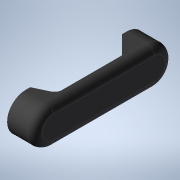
# Autodesk Inventor part: controlbox_handvat
Saved by Autodesk Inventor 2020 (Build 240168000, 168)
## iProperties
Created: 2020-06-02
Part Number: controlbox_handvat
Material: Generic
Document SubType Name: Modeling
Designer: Gebruiker
Density: 1 g/cm^3
Appearance: Default
Author: Gebruiker
Autodesk Inventor part; units mm, degrees
ref_plane "YZ Plane" through (0, 0, 0) normal (1, 0, 0) x (0, 1, 0)
ref_plane "XZ Plane" through (0, 0, 0) normal (0, 1, 0) x (-1, 0, 0)
ref_plane "XY Plane" through (0, 0, 0) normal (0, 0, 1) x (1, 0, 0)
sketch "Sketch1" plane through (0, 0, 0) normal (1, 0, 0) x (0, 1, 0)
  line L0 (10, 37.5) -> (-10, 37.5)
  line L1 (-10, 37.5) -> (-10, -37.5)
  line L2 (-10, -37.5) -> (10, -37.5)
  line L3 (10, -37.5) -> (10, 37.5)
  line L4 (10, 37.5) -> (-10, -37.5) construction
  line L5 (-10, 37.5) -> (10, -37.5) construction
  circle A0 centre (0, 27.5) radius 10
  circle A1 centre (0, -27.5) radius 10
  point P0 (0, 0)
  point P1 (10, -27.5)
  point P2 (10, 27.5)
  point P3 (-10, 27.5)
  point P4 (-10, -27.5)
  dimension "d0" = 20
  dimension "d1" = 75
  dimension "d2" = 20
  dimension "d3" = 20
  dimension "d4" = 55
  constraints: 12 end point, 2 centre point, 2 midpoint, 2 parallel, 1 horizontal, 1 perpendicular, 1 tangent
  measures "d0" distance of L2.end L1.end
  measures "d1" distance of L1.end L0.end
  measures "d2" diameter of A0
  measures "d3" diameter of A1
  measures "d4" distance of A1.centre A0.centre
extrude "Extrusion1" add sketch "Sketch1" against normal blind 15 contours A0 | L3 A1 L1 A0 | A1
sketch "Sketch2" plane through (0, -10, -27.5) normal (0, -1, 0) x (1, 0, 0)
  line L0 (-15, 55) -> (-15, 0) projected
  line L1 (-15, 52.5125) -> (-5.0401, 47.8284)
  line L2 (-5.0401, 47.8284) -> (-5.0401, 7.1716)
  line L3 (-5.0401, 7.1716) -> (-15, 2.4875)
  line L4 (-15, 0) -> (-15, -10) projected
  line L5 (0, 55) -> (0, 65) construction
  line L6 (0, 65) -> (-5.0401, 47.8284) construction
  line L7 (0, -10) -> (0, 0) construction
  line L8 (-5.0401, 7.1716) -> (0, -10) construction
  point P0 (0, 27.5)
  point P1 (-15, 2.4875)
  constraints: 10 end point, 2 equal length, 2 point on line, 1 parallel
extrude "Extrusion2" cut sketch "Sketch2" against normal blind 20
fillet "Fillet1" radius 4 6 edges at (0, -10, 0) (0, 0, -37.5) (0, 10, 0) (0, 0, 37.5) (-5.0401, 0, -20.3284) (-5.0401, 0, 20.3284)
body "Solid1"
